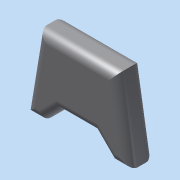
# Autodesk Inventor part: RUCBase
Saved by Autodesk Inventor 2011 SP1 (Build 150282100, 282)
## iProperties
Created: 2011-08-14
Part Number: RUCBase
Document SubType Name: Modeling
Designer: dgitz
Density: 1 g/cm^3
Author: dgitz
Autodesk Inventor part; units mm, degrees
ref_plane "YZ Plane" through (0, 0, 0) normal (1, 0, 0) x (0, 1, 0)
ref_plane "XZ Plane" through (0, 0, 0) normal (0, 1, 0) x (-1, 0, 0)
ref_plane "XY Plane" through (0, 0, 0) normal (0, 0, 1) x (1, 0, 0)
sketch "Sketch1" plane through (0, 0, 0) normal (0, 0, 1) x (1, 0, 0)
  line L0 (-76.2, -49.5971) -> (-57.15, 64.7029)
  line L1 (-57.15, 64.7029) -> (57.15, 64.7029)
  line L2 (57.15, 64.7029) -> (76.2, -49.5971)
  line L3 (-50.8, -49.5971) -> (-25.4, -24.1971)
  line L4 (-25.4, -24.1971) -> (25.4, -24.1971)
  line L5 (25.4, -24.1971) -> (50.8, -49.5971)
  line L6 (76.2, -49.5971) -> (50.8, -49.5971)
  line L7 (-50.8, -49.5971) -> (-76.2, -49.5971)
  point P0 (0, 0)
  dimension "d0" = 152.4
  dimension "d1" = 76.2
  dimension "d3" = 114.3
  dimension "d6" = 67.0095
  dimension "d7" = 114.3
  dimension "d8" = 25.4
  dimension "d9" = 50.8
  dimension "d10" = 25.4
  dimension "d11" = 50.8
  dimension "d12" = 25.4
  constraints: 16 end point, 4 parallel, 3 equal length, 1 horizontal
  measures "d0" distance of L2.end L0.start
  measures "d1" horizontal distance of point (0, 0) L0.start
  measures "d3" distance of L1.end L0.end
  measures "d6" distance from line of point (0, 0) L2
  measures "d7" distance between parallel lines of L7 L1
  measures "d8" distance between parallel lines of L7 L4
  measures "d9" horizontal distance of L3.end L0.start
  measures "d10" distance of L0.start L3.start
  measures "d11" distance of L4.end L3.end
  measures "d12" horizontal distance of point (0, 0) L3.end
extrude "Extrusion1" add sketch "Sketch1" along normal blind 38.1
fillet "Fillet1" radius 12.7 16 edges at (-38.1, -36.8971, 38.1) (-63.5, -49.5971, 38.1) (-66.675, 7.5529, 38.1) (0, -24.1971, 38.1) (38.1, -36.8971, 38.1) (63.5, -49.5971, 38.1) (66.675, 7.5529, 38.1) (0, 64.7029, 38.1) (66.675, 7.5529, 0) (0, 64.7029, 0) (-66.675, 7.5529, 0) (-63.5, -49.5971, 0) (-38.1, -36.8971, 0) (0, -24.1971, 0) (38.1, -36.8971, 0) (63.5, -49.5971, 0)
body "Solid1"
